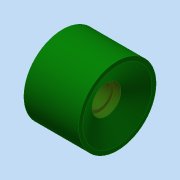
# Autodesk Inventor part: LongboardWheel_RI
Saved by Autodesk Inventor 2015 SP1 (Build 190203100, 203)
## iProperties
Created: 2015-06-17
Part Number: LongboardWheel_RI
Material: Nylon 6/6
Document SubType Name: Modeling
Designer: YOUR_NAME_HERE
Density: 1.13 g/cm^3
Appearance: Dark Green
Author: YOUR_NAME_HERE
Autodesk Inventor part; units mm, degrees
ref_plane "YZ Plane" through (0, 0, 0) normal (1, 0, 0) x (0, 1, 0)
ref_plane "XZ Plane" through (0, 0, 0) normal (0, 1, 0) x (-1, 0, 0)
ref_plane "XY Plane" through (0, 0, 0) normal (0, 0, 1) x (1, 0, 0)
sketch "Sketch1" plane through (0, 0, 0) normal (1, 0, 0) x (0, 1, 0)
  circle A0 centre (0, 0) radius 37.5
  dimension "d0" = 75
  constraints: 1 centre point, 1 coincident
  measures "d0" diameter of A0
extrude "Extrusion1" add sketch "Sketch1" along normal mid plane 53
sketch "Sketch2" plane through (26.5, 0, 0) normal (1, 0, 0) x (0, 0, -1)
  circle A0 centre (0, 0) radius 14
  dimension "d3" = 28
  constraints: 1 centre point, 1 coincident
  measures "d3" diameter of A0
extrude "Extrusion2" cut sketch "Sketch2" against normal blind 17.5
ref_plane "Work Plane1" through (16, 0, 0) normal (1, 0, 0) x (0, 0, -1)
sketch "Sketch3" plane through (0, 0, 0) normal (0, 0, 1) x (1, 0, 0)
  line L0 (-26.5, 37.5) -> (26.5, 37.5) projected
  line L1 (26.5, -37.5) -> (26.5, 37.5) projected
  line L2 (16, 52.5) -> (16, -52.5) projected
  line L3 (26.5, 33.5) -> (-26.5, 33.5)
  line L4 (-26.5, 37.5) -> (-26.5, -37.5) projected
  line L5 (26.5, 14) -> (9, 14) projected
  line L6 (16, 14) -> (26.5, 33.5)
  line L7 (-37.1, 0) -> (37.1, 0) projected
  point P0 (0, 0)
  dimension "d7" = 4
  constraints: 4 end point, 4 point on line, 1 horizontal
  measures "d7" distance between parallel lines of L0 L3
revolve "Revolution1" cut sketch "Sketch3" angle 360 about axis through (-10, 0, 0) along (1, 0, 0) contours L1 L5 L6
sketch "Sketch4" plane through (9, 0, 0) normal (1, 0, 0) x (0, 0, -1)
  circle A0 centre (0, 0) radius 11
  dimension "d9" = 22
  constraints: 1 centre point, 1 coincident
  measures "d9" diameter of A0
extrude "Extrusion3" cut sketch "Sketch4" against normal through all
sketch "Sketch5" plane through (-26.5, 0, 0) normal (-1, 0, 0) x (0, 0, 1)
  circle A0 centre (0, 0) radius 28.5
  circle A1 centre (0, 0) radius 37.5 projected
  dimension "d13" = 9
  constraints: 1 centre point, 1 coincident
  measures "d13" radial gap between concentric circles of A1 A0
ref_plane "Work Plane2" through (-17, 0, 0) normal (1, 0, 0) x (0, 0, -1)
sketch "Sketch6" plane through (0, 0, 0) normal (0, 0, 1) x (1, 0, 0)
  line L0 (-26.5, 28.5) -> (-26.5, -28.5) projected
  line L1 (9, 11) -> (-26.5, 11) projected
  line L2 (-17, 52.5) -> (-17, -52.5) projected
  line L3 (-17, 11) -> (-26.5, 28.5)
  line L4 (-37.1, 0) -> (37.1, 0) projected
  point P0 (0, 0)
  constraints: 2 end point, 2 point on line
revolve "Revolution2" cut sketch "Sketch6" angle 360 about axis through (-10, 0, 0) along (1, 0, 0) contours L3 L1 L0
body "Solid1"
